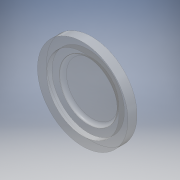
# Autodesk Inventor part: стеклышка
Saved by Autodesk Inventor 2016 (Build 200138000, 138)
## iProperties
Created: 2021-05-08
Part Number: стеклышка
Material: Типовые
Document SubType Name: Modeling
Designer: Лол
Density: 1 g/cm^3
Appearance: Поликарбонат — прозрачный
Author: Лол
Autodesk Inventor part; units mm, degrees
ref_plane "YZ Plane" through (0, 0, 0) normal (1, 0, 0) x (0, 1, 0)
ref_plane "XZ Plane" through (0, 0, 0) normal (0, 1, 0) x (-1, 0, 0)
ref_plane "XY Plane" through (0, 0, 0) normal (0, 0, 1) x (1, 0, 0)
sketch "Эскиз1" plane through (0, 0, 0) normal (0, 0, 1) x (1, 0, 0)
  arc A0 (0, 8) -> (-25, 5) centre (0, -97.6667) ccw
  line L0 (-25, 5) -> (-25, 0)
  line L1 (-30.1076, 0) -> (5.0179, 0) construction
  line L2 (0, -118.9495) -> (0, 30.0301) projected
  line L3 (-20, 0) -> (-20, 3)
  line L4 (-20, 3) -> (-16, 3)
  line L5 (-25, 0) -> (-20, 0)
  line L6 (-16, 3) -> (-16, 5)
  line L7 (0, 8) -> (0, 6.2883)
  arc A1 (0, 6.2883) -> (-16, 5) centre (0, -93.7117) ccw
  point P0 (0, 0)
  point P1 (0, 0)
  point P2 (0, 4.6333)
  dimension "d2" = 5
  dimension "d4" = 25
  dimension "d25" = 3
  dimension "d28" = 16
  dimension "d29" = 20
  dimension "d30" = 100
  dimension "d31" = 2
  dimension "d35" = 8
  constraints: 12 end point, 4 point on circle, 2 centre point, 2 perpendicular, 2 point on line, 2 vertical, 1 collinear, 1 horizontal, 7 other
  measures "d2" distance of L0.start L0.end
  measures "d4" distance of L0.end point (0, 0)
  measures "d25" distance between parallel lines of L1 L4
  measures "d29" distance of the line from the sketch origin of L3
  measures "d30" radius of A1
  measures "d31" distance of L4.end L6.end
  measures "d35" distance from line of L7.start L1
revolve "Вращение1" add sketch "Эскиз1" angle 360 about axis through (0, -10, 0) along (0, 1, 0)
fillet "Сопряжение1" radius 2 1 edges at (16, 5, 0)
